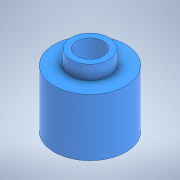
# Autodesk Inventor part: 4mm_Roller_Spacer
Saved by Autodesk Inventor 2021 (Build 250183000, 183)
## iProperties
Created: 2021-03-29
Part Number: 4mm_Roller_Spacer
Material: PET Plastic
Document SubType Name: Modeling
Designer: Jorian Brusind
Density: 1.541 g/cm^3
Appearance: Cyan
Author: Jorian Brusind
Autodesk Inventor part; units mm, degrees
ref_plane "YZ Plane" through (0, 0, 0) normal (1, 0, 0) x (0, 1, 0)
ref_plane "XZ Plane" through (0, 0, 0) normal (0, 1, 0) x (-1, 0, 0)
ref_plane "XY Plane" through (0, 0, 0) normal (0, 0, 1) x (1, 0, 0)
sketch "Sketch4" plane through (0, 0, 0) normal (0, 1, 0) x (-1, 0, 0)
  circle A0 centre (0, 0) radius 7.5
  circle A1 centre (0, 0) radius 2.75
  dimension "d19" = 15
  dimension "d20" = 5.5
  constraints: 2 centre point, 2 coincident
  measures "d19" diameter of A0
  measures "d20" diameter of A1
extrude "Extrusion4" add sketch "Sketch4" along normal blind 12
sketch "Sketch5" plane through (0, 12, 0) normal (0, 1, 0) x (1, 0, 0)
  circle A0 centre (0, 0) radius 2.75 projected
  circle A1 centre (0, 0) radius 2.75
  circle A2 centre (0, 0) radius 4
  dimension "d23" = 5.5
  dimension "d24" = 8
  constraints: 2 centre point, 2 coincident
  measures "d23" diameter of A1
  measures "d24" diameter of A2
extrude "Extrusion5" add sketch "Sketch5" along normal blind 3
body "Solid2"
